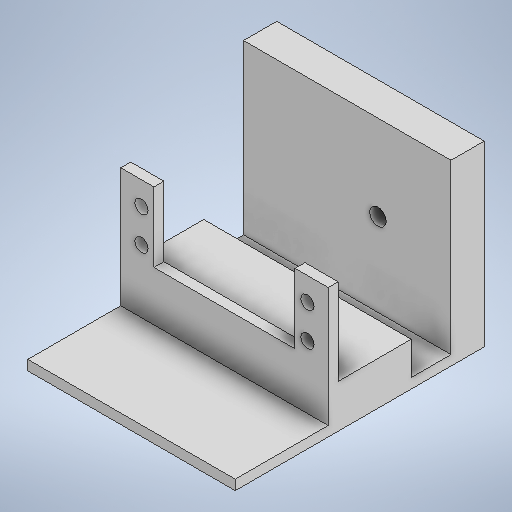
# Autodesk Inventor part: Mounting2
Saved by Autodesk Inventor 2025.3 (Build 293356000, 356)
## iProperties
Created: 2025-10-08
Part Number: Mounting2
Material: Genérico
Document SubType Name: Modeling
Designer: Skuarex
Density: 1 g/cm^3
Appearance: Valor por defecto
Author: Skuarex
Autodesk Inventor part; units mm, degrees
ref_plane "YZ Plane" through (0, 0, 0) normal (1, 0, 0) x (0, 1, 0)
ref_plane "XZ Plane" through (0, 0, 0) normal (0, 1, 0) x (-1, 0, 0)
ref_plane "XY Plane" through (0, 0, 0) normal (0, 0, 1) x (1, 0, 0)
sketch "Boceto1" plane through (0, 0, 0) normal (0, 1, 0) x (-1, 0, 0)
  line L0 (0, 0) -> (-62.5, 0)
  line L1 (-62.5, 0) -> (-62.5, -75)
  line L2 (-62.5, -75) -> (0, -75)
  line L3 (0, -75) -> (0, 0)
  dimension "d0" = 62.5
  dimension "d1" = 75
  constraints: 8 end point, 2 parallel, 1 horizontal, 1 perpendicular
  measures "d0" distance of L2.end L1.end
  measures "d1" distance of L1.end L0.end
extrude "Extrusión1" add sketch "Boceto1" along normal blind 3
sketch "Boceto3" plane through (0, 3, 0) normal (0, 1, 0) x (1, 0, 0)
  line L0 (0, 0) -> (62.5, 0) construction
  line L1 (31.25, 0) -> (31.25, 28) construction
  line L2 (31.25, 28) -> (0, 28)
  line L3 (0, 28) -> (0, 31)
  line L4 (0, 75) -> (0, 0) projected
  line L5 (0, 31) -> (62.5, 31)
  line L6 (62.5, 0) -> (62.5, 75) projected
  line L7 (62.5, 28) -> (31.25, 28)
  line L8 (10, 28) -> (10, 31)
  line L9 (52.5, 28) -> (52.5, 31)
  line L10 (31.25, 31) -> (31.25, 53) construction
  line L11 (31.25, 53) -> (0, 53)
  line L12 (31.25, 53) -> (62.5, 53)
  line L13 (62.5, 75) -> (0, 75) construction
  line L14 (31.25, 75) -> (31.25, 65) construction
  line L15 (62.5, 65) -> (0, 65)
  line L16 (0, 65) -> (0, 75)
  line L17 (62.5, 75) -> (62.5, 65)
  line L18 (62.5, 75) -> (0, 75)
  dimension "d4" = 28
  dimension "d5" = 3
  dimension "d9" = 22
  dimension "d10" = 10
  constraints: 30 end point, 13 point on line, 6 perpendicular, 3 midpoint, 3 vertical, 2 collinear, 1 horizontal, 1 parallel
  measures "d4" distance of L1.start L1.end
  measures "d5" distance of L2.end L3.end
  measures "d9" distance of L10.start L10.end
  measures "d10" distance of L14.start L14.end
extrude "Extrusión2" add sketch "Boceto3" along normal blind 36 contours L2 L3 L5 L8 | L9 L5 L6 L7
extrude "Extrusión3" add sketch "Boceto3" along normal blind 15 contours L2 L8 L5 L9 L7
extrude "Extrusión4" add sketch "Boceto3" along normal blind 10 contours L5 L4 L11 L12 L6
extrude "Extrusión5" add sketch "Boceto3" along normal blind 50.7 contours L4 L18 L6 L15
sketch "Boceto4" plane through (0, 3, -28) normal (0, 0, 1) x (1, 0, 0)
  line L0 (62.5, 0) -> (0, 0) construction
  line L1 (62.5, 0) -> (62.5, 36) construction
  line L2 (52.5, 36) -> (62.5, 36) construction
  line L3 (52.5, 15) -> (52.5, 36) construction
  line L4 (10, 15) -> (52.5, 15) construction
  line L5 (10, 15) -> (10, 36) construction
  line L6 (0, 36) -> (10, 36) construction
  line L7 (0, 0) -> (0, 36) construction
  line L8 (0, 0) -> (0, 22) construction
  line L9 (0, 0) -> (0, 32) construction
  line L10 (0, -3) -> (0, 19) construction
  line L11 (0, 19) -> (62.5, 19) construction
  line L12 (0, -3) -> (0, 29) construction
  line L13 (0, 29) -> (62.5, 29) construction
  line L14 (0, 29) -> (6.25, 29) construction
  line L15 (0, 19) -> (6.25, 19) construction
  line L16 (62.5, 29) -> (56.25, 29) construction
  line L17 (62.5, 19) -> (56.25, 19) construction
  circle A0 centre (6.25, 29) radius 2
  circle A1 centre (6.25, 19) radius 2
  line L18 (62.5, -3) -> (0, -3) construction
  line L19 (31.25, -3) -> (31.25, 50.7118) construction
  circle A2 centre (56.25, 29) radius 2
  circle A3 centre (56.25, 19) radius 2
  dimension "d21" = 22
  dimension "d22" = 32
  dimension "d23" = 6.25
  dimension "d24" = 6.25
  dimension "d25" = 6.25
  dimension "d26" = 4
  dimension "d27" = 4
  constraints: 22 end point, 10 point on line, 4 centre point, 2 coincident, 2 perpendicular, 2 symmetric about line, 1 midpoint, 1 vertical, 2 other
  measures "d21" distance of L10.start L10.end
  measures "d22" distance of L10.start L12.end
  measures "d23" distance of L12.end L14.end
  measures "d24" distance of L10.end L15.end
  measures "d25" distance of L13.end L16.end
  measures "d26" diameter of A0
  measures "d27" diameter of A1
extrude "Extrusión6" cut sketch "Boceto4" against normal blind 20
sketch "Boceto5" plane through (0, 3, -65) normal (0, 0, 1) x (1, 0, 0)
  line L0 (62.5, -3) -> (0, -3) construction
  line L1 (0, -3) -> (0, 25) construction
  line L2 (0, 10) -> (0, 36) construction
  line L3 (0, -3) -> (40.5, -3) construction
  line L4 (40.5, -3) -> (40.5, 25) construction
  circle A0 centre (40.5, 25) radius 2.5
  dimension "d30" = 28
  dimension "d31" = 40.5
  dimension "d32" = 5
  constraints: 6 end point, 2 point on line, 1 centre point, 1 coincident, 1 perpendicular
  measures "d30" distance of L0.end L1.end
  measures "d31" distance of L0.end L3.end
  measures "d32" diameter of A0
extrude "Extrusión7" cut sketch "Boceto5" against normal blind 20
